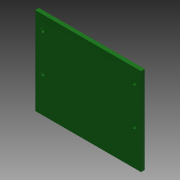
# Autodesk Inventor part: CombinerBoard
Saved by Autodesk Inventor 2014 (Build 180170000, 170)
## iProperties
Created: 2015-04-15
Part Number: CombinerBoard
Material: Generic
Document SubType Name: Modeling
Designer: Owner
Density: 1 g/cm^3
Appearance: Smooth - Dark Forest Green
Author: Owner
Autodesk Inventor part; units mm, degrees
ref_plane "YZ Plane" through (0, 0, 0) normal (1, 0, 0) x (0, 1, 0)
ref_plane "XZ Plane" through (0, 0, 0) normal (0, 1, 0) x (-1, 0, 0)
ref_plane "XY Plane" through (0, 0, 0) normal (0, 0, 1) x (1, 0, 0)
sketch "Sketch1" plane through (0, 0, 0) normal (0, 0, 1) x (1, 0, 0)
  line L0 (15.9308, -18.6059) -> (-31.3132, -18.6059)
  line L1 (-31.3132, -18.6059) -> (-31.3132, 20.3831)
  line L2 (-31.3132, 20.3831) -> (15.9308, 20.3831)
  line L3 (15.9308, 20.3831) -> (15.9308, -18.6059)
  point P0 (0, 0)
  dimension "d0" = 38.989
  dimension "d1" = 47.244
  constraints: 8 end point, 2 parallel, 1 horizontal, 1 perpendicular
  measures "d0" distance of L2.end L0.start
  measures "d1" distance of L1.end L2.end
extrude "Extrusion1" add sketch "Sketch1" along normal blind 1.67
sketch "Sketch2" plane through (0, 0, 1.67) normal (0, 0, 1) x (1, 0, 0)
  line L0 (-31.3132, -18.6059) -> (15.9308, -18.6059) projected
  line L1 (15.9308, -18.6059) -> (15.9308, 20.3831) projected
  line L2 (15.9308, 20.3831) -> (-31.3132, 20.3831) projected
  line L3 (-31.3132, 20.3831) -> (-31.3132, -18.6059) projected
  circle A0 centre (-28.1382, 14.0331) radius 0.7937
  circle A1 centre (12.7558, 14.0331) radius 0.7937
  circle A2 centre (12.7558, -2.7309) radius 0.7937
  circle A3 centre (-28.1382, -2.7309) radius 0.7937
  point P0 (0, 0)
  dimension "d4" = 1.5875
  dimension "d5" = 1.5875
  dimension "d6" = 1.5875
  dimension "d7" = 1.5875
  dimension "d8" = 3.175
  dimension "d9" = 3.175
  dimension "d10" = 3.175
  dimension "d11" = 3.175
  dimension "d12" = 15.875
  dimension "d13" = 15.875
  dimension "d14" = 6.35
  dimension "d15" = 6.35
  constraints: 4 centre point
  measures "d4" diameter of A0
  measures "d5" diameter of A3
  measures "d6" diameter of A2
  measures "d7" diameter of A1
  measures "d8" distance from line of L3 A0.centre
  measures "d9" distance from line of L3 A3.centre
  measures "d10" distance from line of L1 A2.centre
  measures "d11" distance from line of L1 A1.centre
  measures "d12" distance from line of L0 A2.centre
  measures "d13" distance from line of L0 A3.centre
  measures "d14" distance from line of L2 A0.centre
  measures "d15" distance from line of L2 A1.centre
extrude "Extrusion2" cut sketch "Sketch2" against normal up to next contours A0 | A1 | A2 | A3
body "Solid1"
